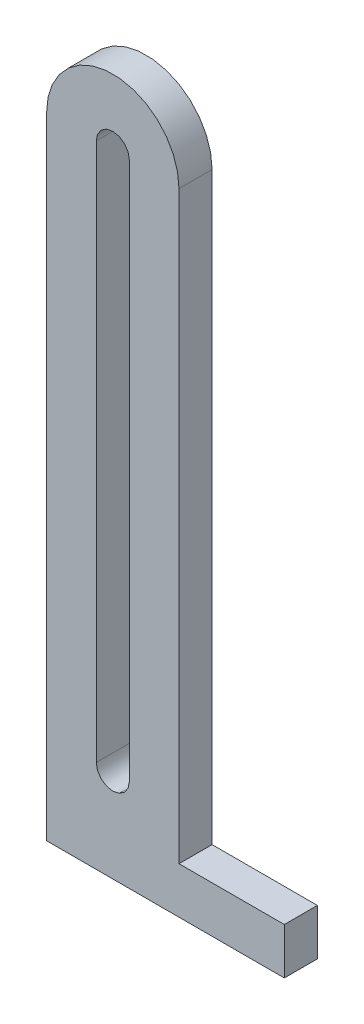
# Autodesk Inventor part: Part10
Saved by Autodesk Inventor 2022 (Build 260153000, 153)
## iProperties
Created: 2021-12-03
Part Number: Part10
Material: Generic
Document SubType Name: Modeling
Designer: alber
Density: 1 g/cm^3
Appearance: Default
Author: alber
Autodesk Inventor part; units mm, degrees
ref_plane "YZ Plane" through (0, 0, 0) normal (1, 0, 0) x (0, 1, 0)
ref_plane "XZ Plane" through (0, 0, 0) normal (0, 1, 0) x (-1, 0, 0)
ref_plane "XY Plane" through (0, 0, 0) normal (0, 0, 1) x (1, 0, 0)
ref_plane "Work Plane1" through (-11.8222, -20.0934, 157.0861) normal (0, 0, -1) x (-1, 0, 0)
sketch "Sketch1" plane through (-11.8222, -20.0934, 157.0861) normal (0, 0, -1) x (-1, 0, 0)
  point P0 (-11.8222, 20.0934)
sketch "Sketch2" plane through (-11.8222, -20.0934, 157.0861) normal (0, 0, -1) x (-1, 0, 0)
  line L0 (6.9228, 0) -> (0, 0) projected
  line L1 (6.9228, -7) -> (0, -7) projected
  line L2 (15.9102, -7) -> (15.9102, 88.3356)
  line L3 (35.9102, 88.3356) -> (35.9102, -7)
  arc A0 (28.4102, 88.3356) -> (23.4102, 88.3356) centre (25.9102, 88.3356) ccw
  circle A1 centre (25.9102, 6.9974) radius 2.5
  line L4 (28.4102, 6.9974) -> (28.4102, 88.3356)
  line L5 (23.4102, 88.3356) -> (23.4102, 6.9974)
  arc A2 (35.9102, 88.3356) -> (15.9102, 88.3356) centre (25.9102, 88.3356) ccw
  line L6 (6.9228, -7) -> (35.9102, -7)
  line L7 (6.9228, 0) -> (15.9102, 0)
  line L8 (0, 0) -> (0, -7)
  point P0 (-11.8222, 20.0934)
  dimension "d2" = 5
  dimension "d3" = 5
  constraints: 14 end point, 6 point on circle, 3 centre point, 2 perpendicular, 2 point on line, 2 tangent, 1 concentric, 1 parallel, 1 vertical, 2 other
  measures "d2" diameter of A0
  measures "d3" diameter of A1
extrude "Extrusion1" add sketch "Sketch2" along normal blind 5
body "Solid1"
